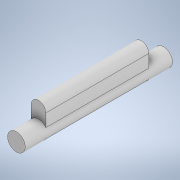
# Autodesk Inventor part: ведущий вал
Saved by Autodesk Inventor 2020 (Build 240168000, 168)
## iProperties
Created: 2023-01-31
Part Number: ведущий вал
Material: Типовые
Document SubType Name: Modeling
Designer: 89160908988
Density: 1 g/cm^3
Appearance: По умолчанию
Author: 89160908988
Autodesk Inventor part; units mm, degrees
ref_plane "YZ Plane" through (0, 0, 0) normal (1, 0, 0) x (0, 1, 0)
ref_plane "XZ Plane" through (0, 0, 0) normal (0, 1, 0) x (-1, 0, 0)
ref_plane "XY Plane" through (0, 0, 0) normal (0, 0, 1) x (1, 0, 0)
sketch "Эскиз4" plane through (0, 0, 0) normal (0, 0, 1) x (1, 0, 0)
  circle A0 centre (0, 0) radius 3
  dimension "d8" = 6
  constraints: 1 centre point, 1 coincident
  measures "d8" diameter of A0
extrude "Выдавливание3" add sketch "Эскиз4" along normal blind 50
sketch "Эскиз5" plane through (0, 0, 0) normal (0, 1, 0) x (-1, 0, 0)
  line L0 (0, 0) -> (0, 25)
  line L1 (-2.5, 42.5) -> (2.5, 42.5)
  line L2 (2.5, 42.5) -> (2.5, 7.5)
  line L3 (2.5, 7.5) -> (-2.5, 7.5)
  line L4 (-2.5, 7.5) -> (-2.5, 42.5)
  line L5 (-2.5, 42.5) -> (2.5, 7.5) construction
  line L6 (2.5, 42.5) -> (-2.5, 7.5) construction
  dimension "d11" = 25
  dimension "d12" = 5
  dimension "d13" = 35
  constraints: 14 end point, 2 midpoint, 2 parallel, 1 horizontal, 1 perpendicular, 1 vertical
  measures "d11" distance of L0.start L0.end
  measures "d12" distance of L2.end L3.end
  measures "d13" distance of L1.end L2.end
extrude "Выдавливание4" cut sketch "Эскиз5" against normal mid plane 50
sketch "Эскиз6" plane through (0, 0, 42.5) normal (0, 0, -1) x (-1, 0, 0)
  point P0 (0, 0)
sketch "Эскиз7" plane through (0, 0, 7.5) normal (0, 0, 1) x (1, 0, 0)
  circle A0 centre (0, 0) radius 3
  line L0 (0, 0) -> (0, 6) construction
  arc A1 (2.5, 1.6583) -> (-2.5, 1.6583) centre (0, 0) ccw projected
  line L1 (2.5, 0) -> (2.5, 6)
  line L2 (-2.5, 6) -> (-2.5, 0)
  arc A2 (-2.5, 0) -> (2.5, 0) centre (0, 0) ccw
  arc A3 (2.5, 6) -> (-2.5, 6) centre (0, 6) ccw
  point P0 (1, 1)
  point P1 (0, 3)
  dimension "d16" = 3
  dimension "d17" = 5
  constraints: 8 end point, 5 point on circle, 4 tangent, 3 centre point, 1 coincident, 1 midpoint, 1 parallel, 1 vertical
  measures "d16" distance of point (0, 3) L0.end
  measures "d17" diameter of A3
extrude "Выдавливание5" add sketch "Эскиз7" along normal blind 35 contours L1 A2 L2 A0 | A0 L2 A3 L1 picked at (0, 1)
